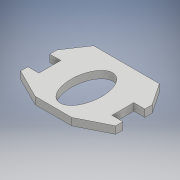
# Autodesk Inventor part: P2-12
Saved by Autodesk Inventor 2017 (Build 210142000, 142)
## iProperties
Created: 2017-02-09
Part Number: P2-12
Material: Generic
Document SubType Name: Modeling
Designer: Schaffel
Density: 1 g/cm^3
Appearance: Default
Author: Schaffel
Autodesk Inventor part; units mm, degrees
ref_plane "YZ Plane" through (0, 0, 0) normal (1, 0, 0) x (0, 1, 0)
ref_plane "XZ Plane" through (0, 0, 0) normal (0, 1, 0) x (-1, 0, 0)
ref_plane "XY Plane" through (0, 0, 0) normal (0, 0, 1) x (1, 0, 0)
sketch "Sketch1" plane through (0, 0, 0) normal (0, 0, 1) x (1, 0, 0)
  line L0 (0, 20) -> (40, 0)
  line L1 (0, 20) -> (0, 30)
  line L2 (0, 30) -> (15, 30)
  line L3 (15, 30) -> (15, 60)
  line L4 (15, 60) -> (0, 60)
  line L5 (0, 60) -> (0, 70)
  line L6 (20, 100) -> (0, 70)
  line L7 (20, 100) -> (110, 100)
  line L8 (130, 70) -> (110, 100)
  line L9 (130, 70) -> (130, 60)
  line L10 (130, 60) -> (115, 60)
  line L11 (115, 60) -> (115, 30)
  line L12 (115, 30) -> (130, 30)
  line L13 (130, 20) -> (130, 30)
  line L14 (90, 0) -> (130, 20)
  line L15 (90, 0) -> (40, 0)
  ellipse E0 centre (65, 45) end of major axis (65, 9) minor radius 20.8465
  point P0 (0, 0)
  constraints: 32 end point, 8 point on line, 5 perpendicular, 2 horizontal, 2 other
extrude "Extrusion1" add sketch "Sketch1" along normal blind 10
body "Solid1"
